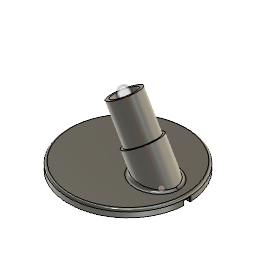
al-base-plate (Autodesk Fusion 360 design; units mm, degrees)
Autodesk Fusion 360 part; units mm, degrees
sketch "Skizze1" plane through (0, 0, 0) normal (0, 0, 1) x (1, 0, 0)
  circle A0 centre (0, 0) radius 80
extrude "Extrusion1" add sketch "Skizze1" along normal blind 10 makes body 1
fillet "Abrundung1" radius 3 1 edges at (-74.5862, -28.9292, 10) on bodies 1
sketch "Skizze2" plane through (0, 0, 0) normal (0, 1, 0) x (1, 0, 0)
  line L0 (45, 0) -> (-5, -86.6025) construction
ref_plane "Arbeitsebene1" through (-5, 0, 86.6025) normal (-0.5, 0, 0.866025) x (0, -1, 0)
sketch "Skizze3" plane through (-5, 0, 86.6025) normal (-0.5, 0, 0.866025) x (0, -1, 0)
  circle A0 centre (0, 0) radius 23
  circle A1 centre (0, 0) radius 20
extrude "Extrusion5" add sketch "Skizze3" against normal blind 110 separate body contours A0 | A1 makes body 2
combine "Kombinieren1" operation add target body 1 tool bodies 2
extrude "Extrusion6" cut sketch "Skizze3" against normal blind 50 bodies 1
fillet "Abrundung2" radius 4 3 edges at (65.7846, 0, 10) (-74.5862, -28.9292, 7) (-71.7892, 27.8444, 10) on bodies 1
sketch "Skizze4" plane through (-5, 0, 86.6025) normal (-0.5, 0, 0.866025) x (0, -1, 0)
  circle A0 centre (0, 0) radius 15.75
extrude "Extrusion7" cut sketch "Skizze4" against normal blind 110 bodies 1
sketch "Skizze5" plane through (0, 0, 0) normal (0, 0, 1) x (1, 0, 0)
  circle A0 centre (0, 0) radius 160
extrude "Extrusion8" cut sketch "Skizze5" against normal blind 110 bodies 1
sketch "Skizze6" plane through (0, 0, 0) normal (0, 0, 1) x (1, 0, 0)
  line L0 (39, 14) -> (51, 14)
  line L1 (51, 14) -> (51, 36)
  line L2 (51, 36) -> (39, 36)
  line L3 (39, 36) -> (39, 14)
  line L4 (39, -36) -> (51, -36)
  line L5 (51, -36) -> (51, -14)
  line L6 (51, -14) -> (39, -14)
  line L7 (39, -14) -> (39, -36)
extrude "Extrusion9" cut sketch "Skizze6" along normal blind 2.5 bodies 1
sketch "Skizze7" plane through (0, 0, 0) normal (0, 0, 1) x (1, 0, 0)
  circle A0 centre (45, 0) radius 21.25
  circle A1 centre (45, 0) radius 28.75
  line L0 (73.75, -3.75) -> (85, -3.75)
  line L1 (85, -3.75) -> (85, 3.75)
  line L2 (85, 3.75) -> (73.75, 3.75)
  line L3 (73.75, 3.75) -> (73.75, -3.75)
  line L4 (16.25, -3.75) -> (33, -3.75)
  line L5 (33, -3.75) -> (33, 3.75)
  line L6 (33, 3.75) -> (16.25, 3.75)
  line L7 (16.25, 3.75) -> (16.25, -3.75)
  line L8 (66.25, -3.75) -> (73.75, -3.75)
  line L9 (73.75, -3.75) -> (73.75, 3.75)
  line L10 (73.75, 3.75) -> (66.25, 3.75)
  line L11 (66.25, 3.75) -> (66.25, -3.75)
extrude "Extrusion10" cut sketch "Skizze7" along normal blind 5 contours A0 A1 L4 L8 L11 | A0 A1 L6 L10 L11 | A1 L8 L10 L11 | A0 L4 L5 L6 | A0 A1 L4 L6 | A1 L6 L7 | A1 L4 L7 | A1 L3 L9 L10 | A1 L3 L8 L9 | L0 L1 L2 L3 L9 picked at (29.929, -0.4186) bodies 1
sketch "Skizze8" plane through (0, 0, 0) normal (0, 0, 1) x (1, 0, 0)
  circle A0 centre (45, 18.5) radius 1.3
  circle A1 centre (45, 31.5) radius 1.3
  circle A2 centre (45, -18.5) radius 1.3
  circle A3 centre (45, -31.5) radius 1.3
extrude "Extrusion11" cut sketch "Skizze8" along normal blind 6 bodies 1
chamfer "Fase1" distance 1 angle 45 3 edges at (79.9121, 3.75, 2.5) (79.9121, -3.75, 2.5) (80, 0, 5) tangent chain off on bodies 1
fillet "Abrundung3" radius 1 4 edges at (25.8931, 3.75, 2.5) (25.8931, -3.75, 2.5) (24.0835, -3.75, 2.5) (24.0835, 3.75, 2.5) on bodies 1
fillet "Abrundung4" radius 2 2 edges at (73.5044, -3.75, 2.5) (73.5044, 3.75, 2.5) on bodies 1
equation "base_plate_diameter = 160 mm" comment "Durchmesser der runden Basis-Platte"
equation "base_plate_height = 10 mm" comment "Höhe der runden Basis-Platte"
equation "base_plate_rounding = 3 mm" comment "Abrundung der oberen Basis-Platte-Kante (Kreis)"
equation "leg_outer_diameter = 46 mm" comment "Aussendurchmesser der Röhre"
equation "ring_inner_diameter = 40 mm" comment "Aussendurchmesser des oberen Röhrensegments (Stufenabsatz)"
equation "ring_extrude_depth = 50 mm" comment "Länge des oberen (dünnen) Röhrensegments / Stufenabsatz"
equation "hole_inner_diameter = 31.5 mm" comment "Innendurchmesser der Röhre (Loch)"
equation "leg_length = 100 mm" comment "Laenge der Röhre"
equation "leg_angle = 120 deg" comment "Winkel des Beines zur XY-Ebene (Innenwinkel an der Platte)"
equation "leg_offset = 45 mm" comment "Abstand des Bein-Fußpunktes vom Plattenmittelpunkt"
equation "leg_plate_rounding = 4 mm" comment "Abrundung der Kante: Bein und Platte (wird bei Solver-Problemen automatisch verkleinert)"
equation "cable_channel_width = 7.5 mm" comment "Breite des unterseitigen Kabelkanals"
equation "cable_channel_depth = 5 mm" comment "Tiefe des unterseitigen Kabelkanals"
equation "clamp_recess_width = 22 mm" comment "Breite der Klemmsteg-Vertiefung quer zum Kanal"
equation "clamp_recess_length = 12 mm" comment "Länge der Klemmsteg-Vertiefung entlang des Kanals"
equation "clamp_recess_depth = 2.5 mm" comment "Tiefe der Klemmsteg-Vertiefung an der Unterseite"
equation "strain_relief_screw_diameter = 2.6 mm" comment "Bohrungsdurchmesser für M3-Zugsicherungsschellen"
equation "strain_relief_screw_depth = 6 mm" comment "Bohrungstiefe für M3-Zugsicherungsschellen"
equation "d19 = base_plate_height"
equation "d22 = base_plate_rounding"
equation "d30 = -( leg_length + base_plate_height )"
equation "d32 = -ring_extrude_depth"
equation "d35 = leg_plate_rounding"
equation "d36 = -leg_length - base_plate_height"
equation "d38 = -( leg_length + base_plate_height )"
equation "d40 = clamp_recess_depth"
equation "d42 = cable_channel_depth"
equation "d44 = strain_relief_screw_depth"
